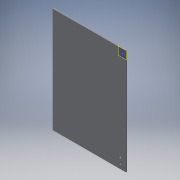
# Autodesk Inventor part: Side Panel
Saved by Autodesk Inventor 2016 (Build 200138000, 138)
## iProperties
Created: 2016-07-16
Part Number: Side Panel
Material: Generic
Document SubType Name: Modeling
Designer: Scott
Density: 1 g/cm^3
Appearance: Default
Author: Scott
Autodesk Inventor part; units mm, degrees
ref_plane "YZ Plane" through (0, 0, 0) normal (1, 0, 0) x (0, 1, 0)
ref_plane "XZ Plane" through (0, 0, 0) normal (0, 1, 0) x (-1, 0, 0)
ref_plane "Work Plane1" through (25.4, 0, 3.81) normal (0, 0, -1) x (-1, 0, 0)
sketch "Sketch1" plane through (25.4, 0, 3.81) normal (0, 0, -1) x (-1, 0, 0)
  circle A0 centre (12.7, 12.7) radius 3.175 projected
  line L0 (0, 0) -> (25.4895, 0) projected
  line L1 (25.4895, 25.4) -> (25.4895, 0) projected
  line L2 (0, 25.4) -> (25.4895, 25.4) projected
  line L3 (0, 0) -> (0, 25.4) projected
  line L4 (0, 25.4) -> (254, 25.4)
  line L5 (254, 25.4) -> (254, -339.6)
  line L6 (254, -339.6) -> (0, -339.6)
  line L7 (0, -339.6) -> (0, 25.4)
  line L8 (0, -339.6) -> (0, -324.36)
  line L9 (0, -324.36) -> (20.32, -324.36)
  line L10 (20.32, -324.36) -> (20.32, -304.04)
  circle A1 centre (20.32, -324.36) radius 3.175
  circle A2 centre (20.32, -304.04) radius 3.175
  point P0 (25.4, 0)
  dimension "d0" = 254
  dimension "d1" = 365
  dimension "d2" = 15.24
  dimension "d3" = 20.32
  dimension "d4" = 20.32
  dimension "d5" = 6.35
  dimension "d6" = 6.35
  constraints: 14 end point, 2 centre point, 2 coincident, 2 parallel, 2 perpendicular, 1 horizontal, 1 point on line, 1 vertical
  measures "d0" distance of L5.end L6.end
  measures "d1" distance of L4.end L5.end
  measures "d2" distance of L6.end L8.end
  measures "d3" distance of L8.end L9.end
  measures "d4" distance of L9.end L10.end
  measures "d5" diameter of A1
  measures "d6" diameter of A2
ref_plane "Work Plane2" through (0, -340.36, 0) normal (0, 0, 1) x (1, 0, 0)
extrude "Extrusion1" add sketch "Sketch1" along normal up to surface (3.81 mm away)
body "Solid1"
